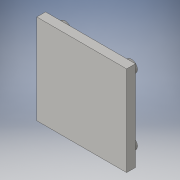
# Autodesk Inventor part: RotatorTop
Saved by Autodesk Inventor 2016 (Build 200138000, 138)
## iProperties
Created: 2016-03-27
Part Number: RotatorTop
Material: Generic
Document SubType Name: Modeling
Designer: mkepler
Density: 1 g/cm^3
Appearance: Default
Author: mkepler
Autodesk Inventor part; units mm, degrees
ref_plane "YZ Plane" through (0, 0, 0) normal (1, 0, 0) x (0, 1, 0)
ref_plane "XZ Plane" through (0, 0, 0) normal (0, 1, 0) x (-1, 0, 0)
ref_plane "XY Plane" through (0, 0, 0) normal (0, 0, 1) x (1, 0, 0)
sketch "Sketch1" plane through (0, 0, 0) normal (0, 1, 0) x (-1, 0, 0)
  line L0 (0, 0) -> (46, 0)
  line L1 (46, 0) -> (46, -46)
  line L2 (46, -46) -> (0, -46)
  line L3 (0, -46) -> (0, 0)
  dimension "d0" = 46
  dimension "d1" = 46
  constraints: 8 end point, 2 parallel, 1 horizontal, 1 perpendicular
  measures "d0" distance of L1.end L2.end
  measures "d1" distance of L0.end L1.end
extrude "Extrusion1" add sketch "Sketch1" along normal blind 4.5
sketch "Sketch2" plane through (0, 4.5, 0) normal (0, 1, 0) x (1, 0, 0)
  circle A0 centre (-40, 6) radius 3.05
  line L0 (-46, 0) -> (-46, 46) projected
  line L1 (-46, 0) -> (0, 0) projected
  circle A1 centre (-40, 40) radius 3.05
  line L2 (0, 46) -> (-46, 46) projected
  circle A2 centre (-6, 6) radius 3.05
  line L3 (0, 0) -> (0, 46) projected
  circle A3 centre (-6, 40) radius 3.05
  dimension "d4" = 6.1
  dimension "d5" = 6
  dimension "d6" = 6
  dimension "d7" = 6.1
  dimension "d8" = 6
  dimension "d9" = 6
  dimension "d10" = 6.1
  dimension "d11" = 6
  dimension "d12" = 6
  dimension "d13" = 6.1
  dimension "d16" = 6
  dimension "d17" = 6
  constraints: 4 centre point
  measures "d4" diameter of A0
  measures "d5" distance from line of L0 A0.centre
  measures "d6" distance from line of L1 A0.centre
  measures "d7" diameter of A1
  measures "d8" distance from line of L0 A1.centre
  measures "d9" distance from line of L2 A1.centre
  measures "d10" diameter of A2
  measures "d11" distance from line of L1 A2.centre
  measures "d12" distance from line of L3 A2.centre
  measures "d13" diameter of A3
  measures "d16" distance from line of L2 A3.centre
  measures "d17" distance from line of L3 A3.centre
extrude "Extrusion2" add sketch "Sketch2" along normal blind 4 contours A0 | A1 | A2 | A3
sketch "Sketch3" plane through (0, 4.5, 0) normal (0, 1, 0) x (1, 0, 0)
  circle A0 centre (-23, 23) radius 12
  point P0 (0, 0)
  dimension "d18" = 24
  constraints: 1 centre point
  measures "d18" diameter of A0
hole "Hole1" at (-23, 4.5, -23) direction (0, -1, 0) diameter 24 depth 1.5
body "Solid1"
